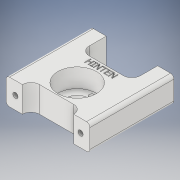
# Autodesk Inventor part: Motorhalterung leicht H
Saved by Autodesk Inventor 2018 (Build 220112000, 112)
## iProperties
Created: 2019-03-03
Part Number: Motorhalterung leicht H
Material: ABS-Kunststoff
Document SubType Name: Modeling
Designer: RedBots
Density: 0.513105 g/cm^3
Appearance: Weiß
Mass: 11 g
Surface Area: 84.958 cm^2
Volume: 21.4381 cm^3
Author: RedBots
Autodesk Inventor part; units mm, degrees
ref_plane "YZ Plane" through (0, 0, 0) normal (1, 0, 0) x (0, 1, 0)
ref_plane "XZ Plane" through (0, 0, 0) normal (0, 1, 0) x (-1, 0, 0)
ref_plane "XY Plane" through (0, 0, 0) normal (0, 0, 1) x (1, 0, 0)
sketch "Skizze2" plane through (0, 0, 0) normal (0, 0, 1) x (1, 0, 0)
  line L0 (0, 0) -> (49, 0)
  line L1 (0, 0) -> (49, 0) construction
  line L2 (49, 0) -> (49, 49)
  line L3 (49, 49) -> (0, 49)
  line L4 (0, 49) -> (0, 0)
  dimension "d16" = 49
  dimension "d18" = 49
  constraints: 10 end point, 2 equal length, 2 horizontal, 2 perpendicular
  measures "d16" distance of L0.start L0.end
  measures "d18" distance of L0.end L2.end
extrude "Extrusion1" add sketch "Skizze2" along normal blind 15
sketch "Skizze3" plane through (0, 0, 15) normal (0, 0, 1) x (1, 0, 0)
  circle A0 centre (24.5, 17) radius 11.25
  line L0 (0, 49) -> (0, 0) construction
  line L1 (0, 17) -> (49, 17) construction
  line L2 (49, 0) -> (49, 49) construction
  line L3 (0, 0) -> (49, 0) construction
  dimension "d72" = 22.5
  dimension "d73" = 17
  constraints: 2 end point, 2 point on line, 1 centre point, 1 coincident, 1 horizontal, 1 midpoint
  measures "d72" diameter of A0
  measures "d73" distance between parallel lines of L3 L1
extrude "Extrusion2" cut sketch "Skizze3" against normal blind 11
sketch "Skizze4" plane through (24.5, 17, 4) normal (0, 0, 1) x (1, 0, 0)
  circle A0 centre (7.3612, -4.25) radius 1.5
  circle A1 centre (0, 8.5) radius 1.5
  circle A2 centre (-7.3612, -4.25) radius 1.5
  line L0 (0, 0) -> (0, 8.5) construction
  line L1 (-24.5, -17) -> (24.5, -17) construction
  circle A3 centre (0, 0) radius 11.25 construction
  line L2 (0, -17) -> (0, 0) construction
  line L3 (0, 0) -> (7.3612, -4.25) construction
  line L4 (0, 0) -> (-7.3612, -4.25) construction
  circle A4 centre (0, 0) radius 6.5
  dimension "d37" = 3
  dimension "d42" = 3
  dimension "d43" = 3
  dimension "d90" = 8.5
  dimension "d91" = 120
  dimension "d92" = 120
  dimension "d93" = 13
  constraints: 8 end point, 4 centre point, 4 coincident, 2 equal length, 2 vertical, 1 midpoint
  measures "d37" diameter of A0
  measures "d42" diameter of A1
  measures "d43" diameter of A2
  measures "d90" distance of L0.start L0.end
  measures "d91" angle of L3 L0
  measures "d92" angle of L0 L4
  measures "d93" diameter of A4
extrude "Extrusion3" cut sketch "Skizze4" against normal up to next
sketch "Skizze9" plane through (0, 49, 0) normal (0, 1, 0) x (1, 0, 0)
  line L0 (24.5, -7.5) -> (43.5, -7.5) construction
  circle A0 centre (5.5, -7.5) radius 1.5
  circle A1 centre (43.5, -7.5) radius 1.5
  line L1 (0, -15) -> (49, -15) construction
  line L2 (24.5, -15) -> (24.5, 0) construction
  line L3 (49, 0) -> (0, 0) construction
  line L4 (5.5, -7.5) -> (24.5, -7.5) construction
  dimension "d58" = 3
  dimension "d89" = 19
  constraints: 7 end point, 3 midpoint, 2 centre point, 2 collinear, 1 coincident, 1 equal radius, 1 horizontal, 1 vertical
  measures "d58" diameter of A0
  measures "d89" distance of L0.start L0.end
extrude "Extrusion6" cut sketch "Skizze9" against normal blind 56
sketch "Skizze12" plane through (0, 0, 0) normal (0, 0, -1) x (-1, 0, 0)
  circle A0 centre (-24.5, 25.5) radius 1.5 projected
  circle A1 centre (-24.5, 25.5) radius 3
  circle A2 centre (-17.1388, 12.75) radius 1.5 projected
  circle A3 centre (-17.1388, 12.75) radius 3
  circle A4 centre (-31.8612, 12.75) radius 1.5 projected
  circle A5 centre (-31.8612, 12.75) radius 3
  point P0 (0, 0)
  dimension "d80" = 6
  dimension "d81" = 6
  dimension "d82" = 6
  constraints: 3 centre point, 3 coincident
  measures "d80" diameter of A1
  measures "d81" diameter of A3
  measures "d82" diameter of A5
extrude "Extrusion8" cut sketch "Skizze12" against normal blind 0.16
chamfer "Fase3" distance 1.5 angle 45 3 edges at (23, 25.5, 0.16) (30.3612, 12.75, 0.16) (15.6388, 12.75, 0.16)
fillet "Rundung2" radius 0.5 3 edges at (23, 25.5, 1.66) (30.3612, 12.75, 1.66) (15.6388, 12.75, 1.66)
sketch "Skizze14" plane through (0, 0, 0) normal (0, 0, -1) x (-1, 0, 0)
  line L0 (-39.5, 49) -> (-9.5, 49)
  line L1 (-9.5, 49) -> (-9.5, 34)
  line L2 (-9.5, 34) -> (-39.5, 34)
  line L3 (-39.5, 34) -> (-39.5, 49)
  line L4 (-49, 49) -> (0, 49) projected
  line L5 (-49, 0) -> (-49, 49) construction
  line L6 (0, 49) -> (0, 0) construction
  line L7 (-39.5, 0) -> (-9.5, 0)
  line L8 (-9.5, 0) -> (-9.5, 5)
  line L9 (-9.5, 5) -> (-39.5, 5)
  line L10 (-39.5, 5) -> (-39.5, 0)
  line L11 (0, 0) -> (-49, 0) projected
  point P0 (-24.5, 49)
  point P1 (-24.5, 0)
  point P2 (-24.5, 0)
  dimension "d95" = 15
  dimension "d96" = 30
  dimension "d101" = 5
  constraints: 16 end point, 6 midpoint, 3 horizontal, 3 parallel, 2 vertical, 1 perpendicular
  measures "d95" distance of L0.end L1.end
  measures "d96" distance between parallel lines of L1 L3
  measures "d101" distance of L7.end L9.start
extrude "Extrusion9" cut sketch "Skizze14" against normal up to next
fillet "Rundung3" radius 5 4 edges at (39.5, 34, 7.5) (9.5, 34, 7.5) (39.5, 5, 7.5) (9.5, 5, 7.5)
fillet "Rundung4" radius 2 4 edges at (49, 24.5, 15) (49, 24.5, 0) (0, 24.5, 0) (0, 24.5, 15)
sketch "Skizze16" plane through (0, 0, 15) normal (0, 0, 1) x (1, 0, 0)
  line L0 (14.5, 34) -> (34.5, 34) construction
  line L1 (24.5, 34) -> (24.5, 28.25) construction
  circle A0 centre (24.5, 17) radius 11.25 projected
  line L2 (18.904, 29.375) -> (18.4388, 29.375)
  line L3 (18.4388, 29.375) -> (18.4388, 31.0881)
  line L4 (18.4388, 31.0881) -> (16.8278, 31.0881)
  line L5 (16.8278, 31.0881) -> (16.8278, 29.375)
  line L6 (16.8278, 29.375) -> (16.3626, 29.375)
  line L7 (16.3626, 29.375) -> (16.3626, 32.875)
  line L8 (16.3626, 32.875) -> (16.8278, 32.875)
  line L9 (16.8278, 32.875) -> (16.8278, 31.5022)
  line L10 (16.8278, 31.5022) -> (18.4388, 31.5022)
  line L11 (18.4388, 31.5022) -> (18.4388, 32.875)
  line L12 (18.4388, 32.875) -> (18.904, 32.875)
  line L13 (18.904, 32.875) -> (18.904, 29.375)
  line L14 (20.8327, 29.375) -> (19.4769, 29.375)
  line L15 (19.4769, 29.375) -> (19.4769, 29.7324)
  line L16 (19.4769, 29.7324) -> (19.9222, 29.7324)
  line L17 (19.9222, 29.7324) -> (19.9222, 32.5176)
  line L18 (19.9222, 32.5176) -> (19.4769, 32.5176)
  line L19 (19.4769, 32.5176) -> (19.4769, 32.875)
  line L20 (19.4769, 32.875) -> (20.8327, 32.875)
  line L21 (20.8327, 32.875) -> (20.8327, 32.5176)
  line L22 (20.8327, 32.5176) -> (20.3874, 32.5176)
  line L23 (20.3874, 32.5176) -> (20.3874, 29.7324)
  line L24 (20.3874, 29.7324) -> (20.8327, 29.7324)
  line L25 (20.8327, 29.7324) -> (20.8327, 29.375)
  line L26 (23.9129, 29.375) -> (23.391, 29.375)
  line L27 (23.391, 29.375) -> (21.8424, 32.3928)
  line L28 (21.8424, 32.3928) -> (21.8424, 29.375)
  line L29 (21.8424, 29.375) -> (21.4084, 29.375)
  line L30 (21.4084, 29.375) -> (21.4084, 32.875)
  line L31 (21.4084, 32.875) -> (22.0693, 32.875)
  line L32 (22.0693, 32.875) -> (23.4789, 30.1039)
  line L33 (23.4789, 30.1039) -> (23.4789, 32.875)
  line L34 (23.4789, 32.875) -> (23.9129, 32.875)
  line L35 (23.9129, 32.875) -> (23.9129, 29.375)
  line L36 (25.4388, 29.375) -> (25.4388, 32.4609)
  line L37 (25.4388, 32.4609) -> (24.2646, 32.4609)
  line L38 (24.2646, 32.4609) -> (24.2646, 32.875)
  line L39 (24.2646, 32.875) -> (27.0782, 32.875)
  line L40 (27.0782, 32.875) -> (27.0782, 32.4609)
  line L41 (27.0782, 32.4609) -> (25.904, 32.4609)
  line L42 (25.904, 32.4609) -> (25.904, 29.375)
  line L43 (25.904, 29.375) -> (25.4388, 29.375)
  line L44 (27.4327, 29.375) -> (27.4327, 32.875)
  line L45 (27.4327, 32.875) -> (29.6224, 32.875)
  line L46 (29.6224, 32.875) -> (29.6224, 32.4609)
  line L47 (29.6224, 32.4609) -> (27.8979, 32.4609)
  line L48 (27.8979, 32.4609) -> (27.8979, 31.5022)
  line L49 (27.8979, 31.5022) -> (29.5061, 31.5022)
  line L50 (29.5061, 31.5022) -> (29.5061, 31.0881)
  line L51 (29.5061, 31.0881) -> (27.8979, 31.0881)
  line L52 (27.8979, 31.0881) -> (27.8979, 29.7891)
  line L53 (27.8979, 29.7891) -> (29.6224, 29.7891)
  line L54 (29.6224, 29.7891) -> (29.6224, 29.375)
  line L55 (29.6224, 29.375) -> (27.4327, 29.375)
  line L56 (32.6374, 29.375) -> (32.1155, 29.375)
  line L57 (32.1155, 29.375) -> (30.5669, 32.3928)
  line L58 (30.5669, 32.3928) -> (30.5669, 29.375)
  line L59 (30.5669, 29.375) -> (30.1329, 29.375)
  line L60 (30.1329, 29.375) -> (30.1329, 32.875)
  line L61 (30.1329, 32.875) -> (30.7938, 32.875)
  line L62 (30.7938, 32.875) -> (32.2034, 30.1039)
  line L63 (32.2034, 30.1039) -> (32.2034, 32.875)
  line L64 (32.2034, 32.875) -> (32.6374, 32.875)
  line L65 (32.6374, 32.875) -> (32.6374, 29.375)
  point P0 (0, 0)
  point P1 (24.5, 31.125)
  point P2 (24.5, 31.125)
  constraints: 2 end point, 2 midpoint, 1 coincident, 1 vertical, 1 vertical alignment, 2 other
emboss "Prägen1" sketch "Skizze16" operation cut depth 1 direction (0, 0, -1) contours L2 L3 L4 L5 L6 L7 L8 L9 L10 L11 L12 L13 | L14 L15 L16 L17 L18 L19 L20 L21 L22 L23 L24 L25 | L26 L27 L28 L29 L30 L31 L32 L33 L34 L35 | L36 L37 L38 L39 L40 L41 L42 L43 | L44 L45 L46 L47 L48 L49 L50 L51 L52 L53 L54 L55 | L56 L57 L58 L59 L60 L61 L62 L63 L64 L65
